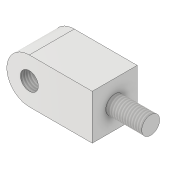
# Autodesk Inventor part: brazos_planetarios1
Saved by Autodesk Inventor 2022 (Build 260153000, 153)
## iProperties
Created: 2019-06-24
Part Number: brazos_planetarios1
Material: Acetal Resin, Black
Document SubType Name: Modeling
Designer: Cristiano
Density: 1.425 g/cm^3
Appearance: Blanco
Author: Cristiano
Autodesk Inventor part; units mm, degrees
ref_plane "YZ Plane" through (0, 0, 0) normal (1, 0, 0) x (0, 1, 0)
ref_plane "XZ Plane" through (0, 0, 0) normal (0, 1, 0) x (-1, 0, 0)
sketch "Boceto1" plane through (0, 0, 0) normal (0, 1, 0) x (-1, 0, 0)
  line L0 (0, 0) -> (35, 0)
  line L1 (47.5, -12.5) -> (47.5, -12.5)
  line L2 (35, -25) -> (0, -25)
  line L3 (0, -25) -> (0, 0)
  line L4 (47.5, -12.5) -> (0, -12.5) construction
  arc A0 (47.5, -12.5) -> (35, 0) centre (35, -12.5) ccw
  arc A1 (35, -25) -> (47.5, -12.5) centre (35, -12.5) ccw
  circle A2 centre (35, -12.5) radius 5
  point P0 (47.5, -25)
  point P1 (47.5, 0)
  dimension "d0" = 25
  dimension "d1" = 47.5
  dimension "d15" = 12.5
  dimension "d16" = 10
  constraints: 10 end point, 4 point on circle, 4 point on line, 4 tangent, 3 centre point, 2 midpoint, 2 parallel, 1 coincident, 1 concentric, 1 horizontal, 1 perpendicular
  measures "d0" distance of L2.end L0.start
  measures "d1" distance of L0.start point (47.5, 0)
  measures "d15" radius of A0
  measures "d16" diameter of A2
ref_plane "Plano de trabajo1" through (0, 0, 0) normal (1, 0, 0) x (0, 0, -1)
extrude "Extrusión3" add sketch "Boceto1" along normal blind 25
sketch "Boceto3" plane through (0, 0, 0) normal (1, 0, 0) x (0, 0, -1)
  circle A0 centre (12.5, 12.5) radius 5
  line L0 (25, 0) -> (25, 25) projected
  line L1 (0, 25) -> (25, 25) projected
  point P0 (0, 0)
  dimension "d19" = 10
  dimension "d20" = 12.5
  dimension "d21" = 12.5
  constraints: 1 centre point
  measures "d19" diameter of A0
  measures "d20" distance from line of L0 A0.centre
  measures "d21" distance from line of L1 A0.centre
extrude "Extrusión4" add sketch "Boceto3" along normal blind 20
thread "Rosca3" size "M10x1.5" class "6g" standard "ANSI Metric M Profile" full length
thread "Rosca4" size "M10x1.5" class "6H" standard "ANSI Metric M Profile" full length
